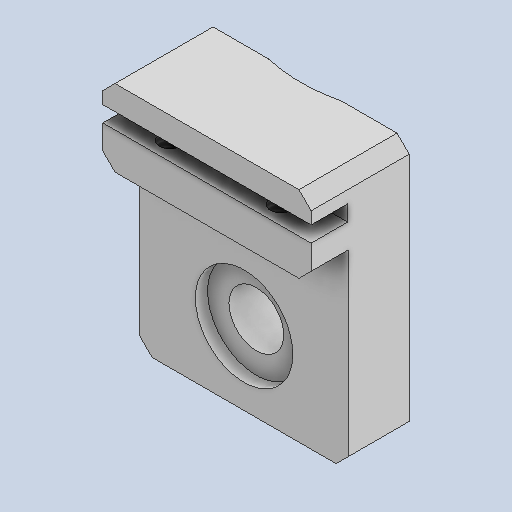
# Autodesk Inventor part: dichroic-mount
Saved by Autodesk Inventor 2024.2 (Build 282272000, 272)
## iProperties
Created: 2021-03-17
Part Number: dichroic-mount
Material: Generic
Document SubType Name: Modeling
Designer: maria
Density: 1 g/cm^3
Appearance: Default
Author: maria
Autodesk Inventor part; units mm, degrees
ref_plane "YZ Plane" through (0, 0, 0) normal (1, 0, 0) x (0, 1, 0)
ref_plane "XZ Plane" through (0, 0, 0) normal (0, 1, 0) x (-1, 0, 0)
ref_plane "XY Plane" through (0, 0, 0) normal (0, 0, 1) x (1, 0, 0)
sketch "Sketch1" plane through (0, 0, 0) normal (0, 0, 1) x (1, 0, 0)
  line L0 (-8.55, 10.5) -> (8.55, 10.5)
  line L1 (8.55, 10.5) -> (8.55, -10.5)
  line L2 (8.55, -10.5) -> (-8.55, -10.5)
  line L3 (-8.55, -10.5) -> (-8.55, 10.5)
  point P0 (0, 0)
  dimension "LENGTH" = 17.1
  dimension "WIDTH" = 21
  dimension "d2" = 10.5
  dimension "d3" = 8.55
  constraints: 8 end point, 2 parallel, 1 horizontal, 1 perpendicular
  measures "LENGTH" distance of L0.start L0.end
  measures "WIDTH" distance of L0.end L1.end
  measures "d2" distance from line of point (0, 0) L0
  measures "d3" distance from line of L1 point (0, 0)
extrude "Extrusion1" add sketch "Sketch1" along normal blind 5
sketch "Sketch4" plane through (0, 0, 5) normal (0, 0, 1) x (1, 0, 0)
  line L0 (-8.55, -10.5) -> (8.55, -10.5) projected
  point P0 (0, 0)
  point P1 (0, -4.5)
  dimension "d16" = 0
  dimension "d17" = 6
  measures "d16" horizontal distance of point (0, 0) point (0, -4.5)
  measures "d17" distance from line of L0 point (0, -4.5)
hole "Hole1" at (0, -4.5, 5) direction (0, 0, -1) diameter 4.5 depth 5 counterbore diameter 8 counterbore depth 1 clearance for "Socket Head Cap Screw" size "#8" standard "Ansi Unified Screw Threads"
sketch "Sketch2" plane through (0, 0, 5) normal (0, 0, 1) x (1, 0, 0)
  line L0 (-8.55, 10.5) -> (8.55, 10.5)
  line L1 (8.55, 10.5) -> (8.55, 4.2)
  line L2 (8.55, 4.2) -> (-8.55, 4.2)
  line L3 (-8.55, 4.2) -> (-8.55, 10.5)
  line L4 (8.55, 6.5) -> (8.55, 5.2)
  line L5 (-8.55, 5.2) -> (-8.55, 6.5)
  point P0 (0, 0)
  dimension "d6" = 10.5
  dimension "d7" = 6.3
  dimension "d8" = 8.55
  dimension "d18" = 17.1
  dimension "d20" = 17.1
  constraints: 12 end point, 3 parallel, 1 horizontal, 1 perpendicular
  measures "d6" distance from line of point (0, 0) L0
  measures "d7" distance of L2.end L0.start
  measures "d8" distance from line of L3 point (0, 0)
  measures "d18" distance of L0.start L0.end
  measures "d20" distance of L5.end L4.start
extrude "Extrusion2" add sketch "Sketch2" along normal blind 14.05
sketch "Sketch7" plane through (0, 0, 19.05) normal (0, 0, 1) x (1, 0, 0)
  line L0 (8.55, 8.5) -> (-8.55, 8.5)
  line L1 (-8.55, 8.5) -> (-8.55, 7.2)
  line L2 (-8.55, 7.2) -> (8.55, 7.2)
  line L3 (8.55, 7.2) -> (8.55, 8.5)
  line L4 (8.55, 4.2) -> (8.55, 10.5) projected
  line L5 (-8.55, 4.2) -> (8.55, 4.2) projected
  line L6 (8.55, 10.5) -> (-8.55, 10.5)
  line L7 (-8.55, 10.5) -> (-8.55, 4.2)
  line L8 (-8.55, 4.2) -> (8.55, 4.2)
  line L9 (8.55, 4.2) -> (8.55, 10.5)
  line L10 (8.55, 10.5) -> (-8.55, 10.5) projected
  point P0 (0, 0)
  point P1 (-8.55, 4.2)
  point P2 (8.55, 8.5)
  point P3 (8.55, 10.5)
  dimension "d53" = 0
  dimension "d54" = 17.1
  dimension "d55" = 1.3
  dimension "d56" = 3
  dimension "d59" = 0
  dimension "d60" = 0
  dimension "d61" = 0
  dimension "d62" = 0
  constraints: 16 end point, 4 parallel, 2 horizontal, 2 perpendicular
  measures "d53" distance between parallel lines of L4 L3
  measures "d54" distance of L0.start L0.end
  measures "d55" distance of L0.end L1.end
  measures "d56" distance between parallel lines of L5 L2
  measures "d59" distance between parallel lines of L3 L9
  measures "d60" distance between parallel lines of L1 L7
  measures "d61" distance between parallel lines of L10 L6
  measures "d62" distance between parallel lines of L5 L8
extrude "Extrusion6" cut sketch "Sketch7" against normal blind 11 contours L0 L7 L6 L4 | L4 L5 L7 L2
extrude "Extrusion5" cut sketch "Sketch7" against normal blind 14 contours L3 L2 L1 L0
sketch "Sketch5" plane through (-8.55, 4.2, 5) normal (0, -1, 0) x (1, 0, 0)
  line L0 (0, 0) -> (0, 3.05) projected
  line L1 (17.1, 0) -> (17.1, 3.05) projected
  line L2 (17.1, 3.05) -> (0, 3.05) projected
  point P0 (8.55, -5)
  point P1 (4, 1.55)
  point P2 (13.1, 1.55)
  point P3 (0, 0.05)
  dimension "d34" = 0
  dimension "d36" = 4
  dimension "d37" = 4
  dimension "d66" = 1.5
  measures "d34" vertical distance of point (13.1, 1.55) point (4, 1.55)
  measures "d36" distance from line of L0 point (4, 1.55)
  measures "d37" distance from line of L1 point (13.1, 1.55)
  measures "d66" vertical distance of point (4, 1.55) point (0, 0.05)
hole "Hole2" at (-4.55, 4.2, 6.55) at (4.55, 4.2, 6.55) direction (0, 1, 0) diameter 1.6942 depth 3 thread size "2-56 UNC" class "2B" standard "ANSI Unified Screw Threads"
sketch "Sketch6" plane through (0, 0, 0) normal (0, 0, -1) x (-1, 0, 0)
  line L0 (5.5, -4.5) -> (4.5, -4.5) construction
  line L1 (5.5, -3.45) -> (4.5, -3.45)
  line L2 (4.5, -5.55) -> (5.5, -5.55)
  arc A0 (5.5, -5.55) -> (5.5, -3.45) centre (5.5, -4.5) ccw
  arc A1 (4.5, -3.45) -> (4.5, -5.55) centre (4.5, -4.5) ccw
  circle A2 centre (0, -4.5) radius 2.25 projected
  point P0 (0, 0)
  point P1 (-5, -4.5)
  point P2 (5, -4.5)
  dimension "d38" = 1
  dimension "d39" = 1.05
  dimension "d40" = 0
  dimension "d41" = 0
  dimension "d42" = 5
  dimension "d43" = 5
  constraints: 8 end point, 4 point on circle, 4 tangent, 2 centre point, 1 horizontal, 1 midpoint, 1 parallel
  measures "d38" distance of L0.start L0.end
  measures "d39" radius of A1
  measures "d40" vertical distance of point (-5, -4.5) point (5, -4.5)
  measures "d41" vertical distance of A2.centre point (-5, -4.5)
  measures "d42" distance of A2.centre point (5, -4.5)
  measures "d43" distance of A2.centre point (-5, -4.5)
hole "Hole3" at (5, -4.5, 0) direction (0, 0, 1) diameter 2.1 depth 2.1
extrude "Extrusion4" cut sketch "Sketch6" against normal blind 2.1 contours A0 L2 A1 L1
chamfer "Chamfer1" distance 1 angle 45 6 edges at (-8.55, 4.2, 6.525) (8.55, 4.2, 6.525) (8.55, 10.5, 4.025) (-8.55, 10.5, 4.025) (8.55, -10.5, 2.5) (-8.55, -10.5, 2.5)
sketch "Sketch8" plane through (-7.55, -10.5, 0) normal (0, -1, 0) x (1, 0, 0)
  circle A0 centre (7.55, -12.35) radius 12.7
  point P0 (7.55, 0)
  dimension "d70" = 0
  dimension "d71" = 12.35
  dimension "d72" = 25.4
  constraints: 1 centre point
  measures "d70" horizontal distance of A0.centre point (7.55, 0)
  measures "d71" distance of point (7.55, 0) A0.centre
  measures "d72" diameter of A0
extrude "Extrusion7" cut sketch "Sketch8" against normal up to surface (21 mm away)
equation "\"d2\" = 0.5 * WIDTH"
equation "\"d3\" = 0.5 * LENGTH"
equation "\"d6\" = 0.5 * WIDTH"
equation "\"d8\" = 0.5 * LENGTH"
equation "\"d18\" = LENGTH"
equation "\"d20\" = LENGTH"
equation "\"d23\" = BEAM_HEIGHT - d4"
equation "\"d54\" = LENGTH"
equation "\"d55\" = DICHROIC_THICKNESS + TOLERANCE"
equation "\"TOLERANCE\" = 0.125"
equation "\"BEAM_HEIGHT\" = 19.05"
equation "\"d4\" = 5"
equation "\"DICHROIC_THICKNESS\" = 1.175"
body "Solid1"
